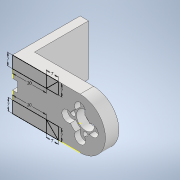
# Autodesk Inventor part: dog_bone_2
Saved by Autodesk Inventor 2020 (Build 240168000, 168)
## iProperties
Created: 2019-05-15
Part Number: dog_bone_2
Material: Generic
Document SubType Name: Modeling
Designer: psrob
Density: 1 g/cm^3
Appearance: Default
Author: psrob
Autodesk Inventor part; units mm, degrees
ref_plane "YZ Plane" through (0, 0, 0) normal (1, 0, 0) x (0, 1, 0)
ref_plane "XZ Plane" through (0, 0, 0) normal (0, 1, 0) x (-1, 0, 0)
ref_plane "XY Plane" through (0, 0, 0) normal (0, 0, 1) x (1, 0, 0)
sketch "Sketch1" plane through (0, 0, 0) normal (0, 0, 1) x (1, 0, 0)
  circle A0 centre (0, 0) radius 2.25 projected
  circle A1 centre (0, 0) radius 15
  circle A2 centre (0, 0) radius 5
  point P0 (0, 0)
  dimension "d0" = 30
  dimension "d1" = 10
  constraints: 2 centre point, 2 coincident
  measures "d0" diameter of A1
  measures "d1" diameter of A2
extrude "Extrusion1" add sketch "Sketch1" along normal blind 8 contours A1
sketch "Sketch2" plane through (0, 0, 8) normal (0, 0, 1) x (1, 0, 0)
  line L0 (-39.9797, 15.0541) -> (-40.0203, -14.9458) projected
  line L1 (-40.0203, -14.9458) -> (-0.0203, -15) projected
  arc A0 (-0.0203, -15) -> (0.0203, 15) centre (0, 0) ccw projected
  line L2 (0.0203, 15) -> (-39.9797, 15.0541) projected
  circle A1 centre (0, 0) radius 5 projected
  circle A2 centre (0, 0) radius 15 projected
  point P0 (0, 0)
extrude "Extrusion2" add sketch "Sketch2" against normal up to surface (8 mm away) contours L2 A2 L1 L0
sketch "Sketch3" plane through (-40.0203, -14.9458, 0) normal (-0.9999991, 0.001354, 0) x (0, 0, 1)
  line L0 (0, 0) -> (0, 30) projected
  line L1 (8, 0) -> (0, 0) projected
  line L2 (8, 30) -> (8, 0) projected
  line L3 (8, 30) -> (0, 30) projected
  line L4 (-86.6334, 30) -> (-86.6334, 0) projected
  line L5 (-86.6334, 0) -> (-46.6334, 0) projected
  line L6 (-46.6334, 0) -> (-46.6334, 30) projected
  line L7 (-46.6334, 30) -> (-86.6334, 30) projected
  line L8 (8, 0) -> (8, 30) projected
  line L9 (8, 0) -> (-32, 0)
  line L10 (-32, 0) -> (-32, 30)
  line L11 (-32, 30) -> (8, 30)
  line L12 (8, 30) -> (8, 0)
  point P0 (0, 15)
  dimension "d6" = 40
  dimension "d7" = 30
  constraints: 8 end point, 2 parallel, 1 horizontal, 1 perpendicular
  measures "d6" distance of L10.end L11.end
  measures "d7" distance of L9.end L10.end
extrude "Extrusion3" add sketch "Sketch3" along normal blind 5 contours L9 L10 L11 L0 | L0 L3 L2 L1
thicken "Thicken1" operation add thickness 5 both sides no extend neighbours yes toward (0.9999991, -0.001354, 0) faces at (-39.9932, 5.0542, -21.3333)
thicken "Thicken2" operation add thickness 5 both sides no extend neighbours yes toward (0.9999991, -0.001354, 0) faces at (-44.9932, 5.0609, -18.6667)
sketch "Sketch6" plane through (0, 0, 8) normal (0, 0, 1) x (1, 0, 0)
  line L0 (-34.9891, 8.0609) -> (-35.0108, -7.9391) projected
  line L1 (-40.0203, -14.9458) -> (-0.0203, -15) projected
  arc A0 (-0.0203, -15) -> (0.0203, 15) centre (0, 0) ccw projected
  line L2 (0.0203, 15) -> (-39.9797, 15.0541) projected
  line L3 (-40.0203, -14.9458) -> (-39.9797, 15.0541) projected
  circle A1 centre (0, 0) radius 5 projected
  line L4 (-43.004, -2.935) -> (-42.9959, 3.065)
  line L5 (-42.9959, 3.065) -> (-36.9959, 3.0569)
  line L6 (-36.9959, 3.0569) -> (-37.004, -2.9431)
  line L7 (-37.004, -2.9431) -> (-43.004, -2.935)
  line L8 (-40.0108, -7.9391) -> (-39.9891, 8.0609) projected
  line L9 (-43.004, -2.935) -> (-36.9959, 3.0569) construction
  line L10 (-42.9959, 3.065) -> (-37.004, -2.9431) construction
  point P0 (0, 0)
  point P1 (-40, 0.0609)
  dimension "d25" = 6
  dimension "d26" = 6
  constraints: 12 end point, 3 midpoint, 2 parallel, 2 perpendicular
  measures "d25" distance of L4.start L4.end
  measures "d26" distance of L4.end L5.end
extrude "Extrusion6" cut sketch "Sketch6" against normal blind 50 contours L7 L4 L5 L3 | L3 L5 L6 L7
sketch "Sketch10" plane through (0, 0, 8) normal (0, 0, 1) x (1, 0, 0)
  arc A0 (-5.7086, 1.8539) -> (-5.3586, -2.6923) centre (-7.4779, -0.5689) ccw projected
  arc A1 (-2.699, 5.3654) -> (-5.7086, 1.8539) centre (0, 0.0068) ccw projected
  arc A2 (1.8471, 5.7154) -> (-2.699, 5.3654) centre (-0.5756, 7.4847) ccw projected
  arc A3 (5.3587, 2.7058) -> (1.8471, 5.7154) centre (0, 0.0068) ccw projected
  arc A4 (5.7086, -1.8403) -> (5.3587, 2.7058) centre (7.4779, 0.5824) ccw projected
  arc A5 (2.6991, -5.3519) -> (5.7086, -1.8403) centre (0, 0.0068) ccw projected
  arc A6 (-1.8471, -5.7018) -> (2.6991, -5.3519) centre (0.5756, -7.4711) ccw projected
  arc A7 (-5.3586, -2.6923) -> (-1.8471, -5.7018) centre (0, 0.0068) ccw projected
  point P0 (0, 0)
  point P1 (5.5531, 2.2723)
  point P2 (5.5469, -2.2873)
  point P3 (-5.3609, -2.6945)
  point P4 (-2.2873, -5.5469)
  point P5 (-2.6963, 5.36)
  point P6 (-5.7066, 1.8532)
  point P7 (2.2873, 5.5469)
ref_plane "Work Plane1" through (-10.5142, -10.5142, 4.75) normal (0, 0, -1) x (0.001354, 0.9999991, 0)
extrude "Extrusion8" cut sketch "Sketch10" against normal up to surface (3.25 mm away)
thicken "Thicken3" operation add thickness 0.25 both sides no extend neighbours yes toward (0.5452549, 0.8382703, 0) faces at (3.2715, 5.0364, 5.8333) (5.7238, 3.0161, 5.8333) (-2.8615, 5.5418, 5.8333) (-3.0463, 5.1759, 6.9167) (-5.7237, -3.0026, 5.8333) (-5.1692, -3.0395, 6.9167) (3.0094, -5.717, 5.8333) (5.4162, -2.575, 5.8333)
sketch "Sketch11" plane through (-0.5756, 7.4847, 4.75) normal (0, 0, 1) x (0.0767503, -0.9970503, 0)
  circle A0 centre (7.5068, -0.0005) radius 5.35
  circle A1 centre (7.5068, -0.0005) radius 5 projected
  arc A2 (4.8279, 5.65) -> (1.85, 2.6721) centre (7.5, 0) ccw projected
  arc A3 (1.85, 2.6721) -> (1.85, -2.6721) centre (0, 0) ccw projected
  arc A4 (1.85, -2.6721) -> (4.8279, -5.65) centre (7.5, 0) ccw projected
  arc A5 (4.8279, -5.65) -> (10.1721, -5.65) centre (7.5, -7.5) ccw projected
  arc A6 (10.1721, -5.65) -> (13.15, -2.6721) centre (7.5, 0) ccw projected
  arc A7 (13.15, -2.6721) -> (13.15, 2.6721) centre (15, 0) ccw projected
  arc A8 (13.15, 2.6721) -> (10.1721, 5.65) centre (7.5, 0) ccw projected
  arc A9 (10.1721, 5.65) -> (4.8279, 5.65) centre (7.5, 7.5) ccw projected
  circle A10 centre (7.5, 7.5) radius 1.5
  circle A11 centre (15, 0) radius 1.5
  circle A12 centre (7.5, -7.5) radius 1.5
  circle A13 centre (0, 0) radius 1.5
  dimension "d48" = 10.7
  dimension "d49" = 3
  dimension "d50" = 3
  dimension "d51" = 3
  dimension "d52" = 3
  constraints: 5 centre point, 5 coincident
  measures "d48" diameter of A0
  measures "d49" diameter of A10
  measures "d50" diameter of A11
  measures "d51" diameter of A12
  measures "d52" diameter of A13
extrude "Extrusion9" cut sketch "Sketch11" against normal blind 10 contours A0 | A1 | A10 | A11 | A12 | A13
sketch "Sketch15" plane through (0, 0, 8) normal (0, 0, 1) x (1, 0, 0)
  arc A0 (-3.0978, 5.435) -> (-5.8384, 2.2373) centre (0, 0.0068) ccw projected
  arc A1 (2.2306, 5.8452) -> (-3.0978, 5.435) centre (-0.5756, 7.4847) ccw projected
  arc A2 (5.4283, 3.1046) -> (2.2306, 5.8452) centre (0, 0.0068) ccw projected
  arc A3 (5.8384, -2.2238) -> (5.4283, 3.1046) centre (7.4779, 0.5824) ccw projected
  arc A4 (3.0978, -5.4215) -> (5.8384, -2.2238) centre (0, 0.0068) ccw projected
  arc A5 (-2.2305, -5.8316) -> (3.0978, -5.4215) centre (0.5756, -7.4711) ccw projected
  arc A6 (-5.4282, -3.0911) -> (-2.2305, -5.8316) centre (0, 0.0068) ccw projected
  arc A7 (-5.8384, 2.2373) -> (-5.4282, -3.0911) centre (-7.4779, -0.5689) ccw projected
  line L0 (-37.004, -2.9431) -> (-40.004, -2.9391) projected
  line L1 (-40.0203, -14.9458) -> (-40.004, -2.9391) projected
  line L2 (-40.0203, -14.9458) -> (-0.0203, -15) projected
  arc A8 (-0.0203, -15) -> (0.0203, 15) centre (0, 0) ccw projected
  line L3 (0.0203, 15) -> (-39.9797, 15.0541) projected
  line L4 (-39.9959, 3.0609) -> (-39.9797, 15.0541) projected
  line L5 (-39.9959, 3.0609) -> (-36.9959, 3.0569) projected
  line L6 (-36.9959, 3.0569) -> (-37.004, -2.9431) projected
  line L7 (-39.9959, 3.0609) -> (-39.9797, 15.0541) projected
  line L8 (-39.9797, 15.0541) -> (-19.9797, 15.0541)
  line L9 (-19.9797, 15.0541) -> (-19.9797, 8.0541)
  line L10 (-19.9797, 8.0541) -> (-39.9797, 8.0541)
  line L11 (-39.9797, 8.0541) -> (-39.9797, 15.0541)
  line L12 (-40.0203, -14.9458) -> (-20.0203, -14.9458)
  line L13 (-20.0203, -14.9458) -> (-20.0203, -7.9458)
  line L14 (-20.0203, -7.9458) -> (-40.0203, -7.9458)
  line L15 (-40.0203, -7.9458) -> (-40.0203, -14.9458)
  line L16 (-19.9797, 8.0541) -> (-12.9797, 8.0541)
  line L17 (-12.9797, 8.0541) -> (-12.9797, 15.0541)
  line L18 (-12.9797, 15.0541) -> (-19.9797, 15.0541)
  line L19 (-19.9797, 15.0541) -> (-19.9797, 8.0541)
  line L20 (-20.0203, -7.9458) -> (-13.0203, -7.9458)
  line L21 (-13.0203, -7.9458) -> (-13.0203, -14.9458)
  line L22 (-13.0203, -14.9458) -> (-20.0203, -14.9458)
  line L23 (-20.0203, -14.9458) -> (-20.0203, -7.9458)
  line L24 (-19.9797, 8.0541) -> (-12.9797, 15.0541)
  line L25 (-20.0203, -7.9458) -> (-13.0203, -14.9458)
  point P0 (0, 0)
  dimension "d69" = 20
  dimension "d70" = 7
  dimension "d71" = 20
  dimension "d72" = 7
  dimension "d73" = 7
  dimension "d74" = 7
  dimension "d75" = 7
  dimension "d76" = 7
  constraints: 36 end point, 8 parallel, 4 horizontal, 4 perpendicular
  measures "d69" distance of L9.end L10.end
  measures "d70" distance of L8.end L9.end
  measures "d71" distance of L14.end L13.end
  measures "d72" distance of L13.end L12.end
  measures "d73" distance of L18.end L17.end
  measures "d74" distance of L17.end L16.end
  measures "d75" distance of L21.end L22.end
  measures "d76" distance of L20.end L21.end
body "Solid1"
